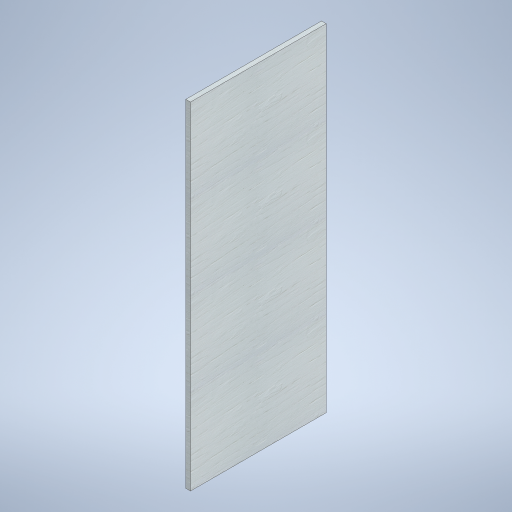
# Autodesk Inventor part: SIDE_CETIN_PART_BOX
Saved by Autodesk Inventor 2023 (Build 270158000, 158)
## iProperties
Created: 2024-02-20
Part Number: SIDE_CETIN_PART_BOX
Material: PVC, Unplasticized
Document SubType Name: Sheet Metal
Designer: vraco
Density: 1.29 g/cm^3
Sheet Metal Rule: Default_mm
Appearance: Wood - Painted White
Author: vraco
Autodesk Inventor part; units mm, degrees
ref_plane "YZ Plane" through (0, 0, 0) normal (1, 0, 0) x (0, 1, 0)
ref_plane "XZ Plane" through (0, 0, 0) normal (0, 1, 0) x (-1, 0, 0)
ref_plane "XY Plane" through (0, 0, 0) normal (0, 0, 1) x (1, 0, 0)
sketch "Sketch1" plane through (0, 0, 0) normal (1, 0, 0) x (0, 1, 0)
  line L0 (0, 101.5) -> (0, -101.5)
  line L1 (-72, 0) -> (432, 0)
  line L2 (0, 72.5) -> (360, 72.5)
  line L3 (360, 72.5) -> (360, -72.5)
  line L4 (360, -72.5) -> (0, -72.5)
  line L5 (0, -72.5) -> (0, 72.5)
  point P0 (0, 0)
  point P1 (0, 0)
  dimension "d0" = 145
  dimension "d1" = 360
  measures "d0" distance of L2.end L3.end
  measures "d1" distance from line of point (0, 0) L3
extrude "Plate1" add sketch "Sketch1" against normal blind 5
equation "\"d2\" = Thickness"
equation "\"BendRadius\" = Thickness"
equation "\"BendReliefWidth\" = Thickness"
equation "\"BendReliefDepth\" = 0.5 * Thickness"
equation "\"TransitionRadius\" = BendRadius"
equation "\"JacobiRadiusSize\" = BendRadius"
equation "\"GapSize\" = Thickness"
equation "\"Thickness\" = 5"
body "Solid1"
